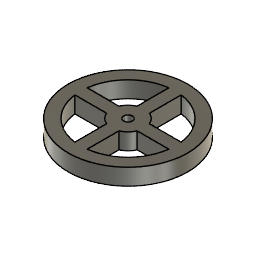
Spoked Wheel (Autodesk Fusion 360 design; units mm, degrees)
Autodesk Fusion 360 part; units mm, degrees
sketch "Sketch1" plane through (0, 0, 0) normal (0, 0, 1) x (1, 0, 0)
  circle A0 centre (0, 0) radius 72.5
  line L0 (0, 0) -> (-170.1079, 0) construction
  arc A1 (-7.5, 57.0088) -> (-57.0088, 7.5) centre (0, 0) ccw
  line L1 (0, 0) -> (0, 73.0172) construction
  line L2 (-57.0088, 7.5) -> (-18.5405, 7.5)
  line L3 (-7.5, 57.0088) -> (-7.5, 18.5405)
  circle A2 centre (0, 0) radius 5
  arc A3 (-7.5, 18.5405) -> (-18.5405, 7.5) centre (0, 0) ccw
  dimension "d2" = 145
  dimension "d9" = 90
  dimension "d10" = 7.5
  dimension "d11" = 7.5
  dimension "d12" = 15
  dimension "d13" = 10
  dimension "d15" = 15
  constraint coincident A0.centre L0.start
  constraint horizontal L0
  constraint parallel L0 L2
  constraint parallel L1 L3
  measures "d2" diameter of A0
  measures "d9" angle of L0 L1
  measures "d10" distance of L0 L2
  measures "d11" distance of L1 L3
  measures "d12" distance of A0 A1
  measures "d13" diameter of A2
  measures "d15" distance of A2 A3
extrude "Extrude1" add sketch "Sketch1" along normal blind 20 contours A0 | A1 L2 L3 A3 | A2
extrude "Extrude2" cut sketch "Sketch1" along normal up to surface (20 mm away) contours A1 L2 L3 A3
extrude "Extrude3" cut sketch "Sketch1" along normal up to surface (20 mm away) draft 1 contours A2
pattern_circular "C-Pattern1" count 4 over 360 about axis through (0, 0, 1.75) along (0, 0, 1) of "Extrude2"
equation "d2 = OverallDiameter"
equation "HubHoleDiameter = 10 mm" comment "Center hole diameter"
equation "HubWallThickness = 15 mm"
equation "NumberOfSPokes = 4"
equation "OverallDiameter = 145 mm" comment "Outside Diameter of the entire part"
equation "PartHeight = 20 mm"
equation "d9 = ( 360 / NumberOfSPokes ) * 1 deg"
equation "d10 = HubWallThickness / 2"
equation "d11 = HubWallThickness / 2"
equation "d12 = HubWallThickness"
equation "d13 = HubHoleDiameter"
equation "d15 = HubWallThickness"
equation "d16 = PartHeight"
equation "HubHoleTaperAngle = 1 deg" comment "Positive values taper outward. Negative inward"
equation "d22 = HubHoleTaperAngle"
equation "d23 = NumberOfSPokes"
named bodies: "Spoked Wheel"
